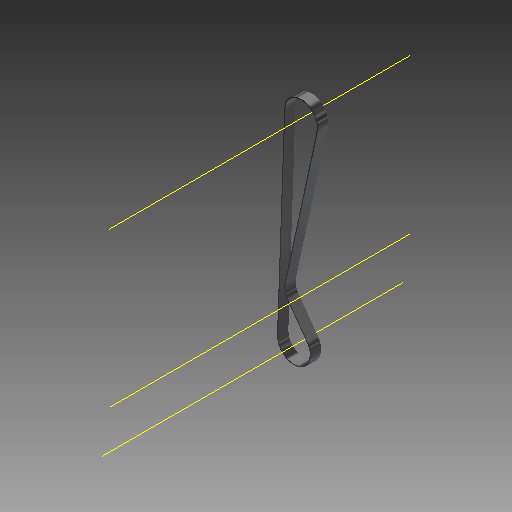
# Autodesk Inventor part: Synchronous Belt
Saved by Autodesk Inventor 2019.4 (Build 234330000, 330)
## iProperties
Created: 2020-01-23
Part Number: Synchronous Belt
Material: Rubber
Document SubType Name: Modeling
Designer: admin
Density: 0.93 g/cm^3
Appearance: Rubber - Black - Version 1.1
Mass: 3.4875 g
Surface Area: 82.5 cm^2
Volume: 3.75 cm^3
CustomPartVersion: 1
Author: admin
Autodesk Inventor part; units mm, degrees
ref_plane "YZ Plane" through (0, 0, 0) normal (1, 0, 0) x (0, 1, 0)
ref_plane "XZ Plane" through (0, 0, 0) normal (0, 1, 0) x (-1, 0, 0)
ref_plane "XY Plane" through (0, 0, 0) normal (0, 0, 1) x (1, 0, 0)
sketch "Sketch Path" plane through (0, 0, 0) normal (0, 0, 1) x (1, 0, 0)
  arc A0 (44.537668, -129.490371) -> (73.337262, -120.736974) centre (60.442743, -130.066194) ccw
  arc A1 (83.039812, 61.123531) -> (51.581722, 65.076727) centre (67.486796, 64.500904) ccw
  arc A2 (51.93378, -82.121723) -> (54.592277, -94.828315) centre (67.486796, -85.499096) ccw
  line L0 (54.592277, -94.828315) -> (73.337262, -120.736974)
  line L1 (44.537668, -129.490371) -> (51.581722, 65.076727)
  line L2 (83.039812, 61.123531) -> (51.93378, -82.121723)
  constraints: 6 end point, 6 point on circle, 3 centre point
ref_plane "Cross Section Plane" through (73.337262, -120.736974, 0) normal (-0.5861722, 0.8101865, 0) x (0, 0, 1)
ref_plane "Work Plane2" through (60.442743, -130.066194, 0) normal (-1, 0, 0) x (0, 0, 1)
ref_plane "Work Plane3" through (67.486796, 64.500904, 0) normal (-0.3272107, -0.9449514, 0) x (0, 0, 1)
ref_plane "Work Plane4" through (67.486796, -85.499096, 0) normal (-0.036735, -0.999325, 0) x (0, 0, 1)
sketch "Cross Section" plane through (73.337262, -120.736974, 0) normal (-0.5861722, 0.8101865, 0) x (0, 0, 1)
  line L0 (-5, 0.5) -> (5, 0.5)
  line L1 (5, 0.5) -> (5, -0.5)
  line L2 (5, -0.5) -> (-5, -0.5)
  line L3 (-5, -0.5) -> (-5, 0.5)
  line L4 (-5, 0) -> (5, 0) construction
  point P0 (0, 0)
  point P1 (0, 0)
  dimension "d0" = 10
  dimension "d4" = 0.5
  dimension "d5" = 0.5
  constraints: 10 end point, 3 midpoint, 2 parallel, 1 coincident, 1 horizontal, 1 perpendicular, 1 other
  measures "d0" distance between parallel lines of L1 L3
  measures "d4" distance between parallel lines of L2 L4
  measures "d5" distance between parallel lines of L4 L0
sweep "Belt" add profiles "Cross Section" path "Sketch Path" path curves L2 A2 L0 A0 L1 A1
equation "\"d0\" = da_B"
equation "\"d4\" = da_a"
equation "\"d5\" = da_a2"
equation "\"da_B\" = 10"
equation "\"da_pb\" = 5"
equation "\"da_a\" = 0.5"
equation "\"da_S\" = 2.65"
equation "\"da_Beta\" = 20deg"
equation "\"da_Ht\" = 1.2"
equation "\"da_H\" = 3.4"
equation "\"da_a2\" = 0.5"
body "Solid1"
